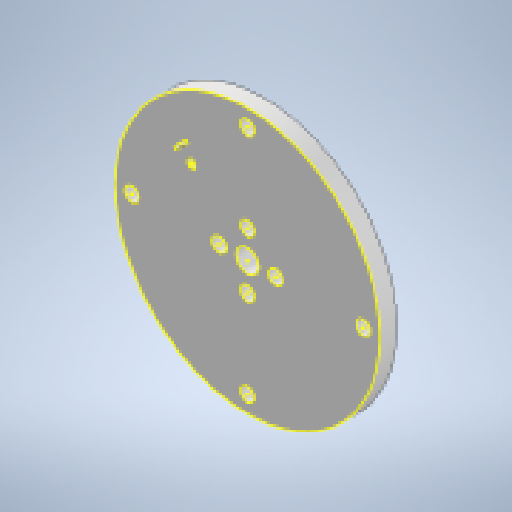
# Autodesk Inventor part: base gear base plate
Saved by Autodesk Inventor 2025 (Build 290162000, 162)
## iProperties
Created: 2025-04-03
Part Number: base gear base plate
Material: 一般
Document SubType Name: Modeling
Designer: gavin
Density: 1 g/cm^3
Appearance: 預設
Author: gavin
Autodesk Inventor part; units mm, degrees
ref_plane "YZ Plane" through (0, 0, 0) normal (1, 0, 0) x (0, 1, 0)
ref_plane "XZ Plane" through (0, 0, 0) normal (0, 1, 0) x (-1, 0, 0)
ref_plane "XY Plane" through (0, 0, 0) normal (0, 0, 1) x (1, 0, 0)
sketch "草圖1" plane through (0, 0, 0) normal (0, 0, 1) x (1, 0, 0)
  circle A0 centre (0, 0) radius 47 projected
  circle A1 centre (40.0673, -8.6957) radius 2.5 construction
  circle A2 centre (-8.6957, -40.0673) radius 2.5 construction
  circle A3 centre (-40.0673, 8.6957) radius 2.5 construction
  circle A4 centre (8.6957, 40.0673) radius 2.5 construction
  circle A5 centre (0, 0) radius 41 construction
  circle A6 centre (41, 0) radius 2.5
  circle A7 centre (0, 41) radius 2.5
  circle A8 centre (-41, 0) radius 2.5
  circle A9 centre (0, -41) radius 2.5
  point P0 (0, 0)
  dimension "d11" = 5
  dimension "d14" = 360
  constraints: 5 centre point, 2 point on circle, 1 coincident, 9 other
  measures "d11" diameter of A6
extrude "擠出1" add sketch "草圖1" along normal blind 6
sketch "草圖3" plane through (0, 0, 6) normal (0, 0, 1) x (1, 0, 0)
  circle A0 centre (0, 0) radius 4
  dimension "d4" = 8
  constraints: 1 centre point, 1 coincident
  measures "d4" diameter of A0
extrude "擠出3" cut sketch "草圖3" against normal through all
sketch "草圖6" plane through (0, 0, 6) normal (0, 0, 1) x (1, 0, 0)
  circle A0 centre (9.4848, 3.1685) radius 2.5 construction
  circle A1 centre (-9.4848, -3.1685) radius 2.5 construction
  circle A2 centre (3.1685, -9.4848) radius 2.5 construction
  circle A3 centre (-3.1685, 9.4848) radius 2.5 construction
  circle A4 centre (0, 0) radius 21 projected
  circle A5 centre (0, 0) radius 4 projected
  circle A6 centre (0, 0) radius 10 construction
  circle A7 centre (10, 0) radius 2.5
  circle A8 centre (0, 10) radius 2.5
  circle A9 centre (-10, 0) radius 2.5
  circle A10 centre (0, -10) radius 2.5
  point P0 (0, 0)
  dimension "d16" = 5
  dimension "d19" = 360
  constraints: 5 centre point, 2 point on circle, 1 coincident, 9 other
  measures "d16" diameter of A7
extrude "擠出5" cut sketch "草圖6" against normal through all contours A7 | A8 | A9 | A10
sketch "草圖10" plane through (0, 0, 6) normal (0, 0, 1) x (1, 0, 0)
  circle A0 centre (-19.8414, 19.8414) radius 1.5
  line L0 (-21.9203, 26.163) -> (-26.163, 21.9203)
  line L1 (-26.163, 21.9203) -> (-25.4983, 21.2556)
  line L2 (-25.4983, 21.2556) -> (-21.2556, 25.4983)
  line L3 (-21.2556, 25.4983) -> (-21.9203, 26.163)
  line L4 (0, 0) -> (-33.234, 33.234) construction
  line L5 (0, 0) -> (18.5986, 0) construction
  circle A1 centre (0, 0) radius 47 projected
  point P0 (-23.377, 23.377)
  dimension "d30" = 3
  dimension "d31" = 0.94
  dimension "d35" = 5
  dimension "d38" = 135
  dimension "d39" = 6
  dimension "d40" = 34
  constraints: 12 end point, 2 parallel, 2 point on line, 1 centre point, 1 horizontal, 1 midpoint, 1 perpendicular, 2 other
  measures "d30" diameter of A0
  measures "d31" distance of L2.end L0.start
  measures "d35" distance from line of L2 A0.centre
  measures "d38" angle of L5 L4
  measures "d39" distance of L0.start L0.end
  measures "d40" distance from line of point (0, 0) L0
extrude "擠出7" cut sketch "草圖10" against normal through all contours A0 | L3 L2 L1 L0
sketch "草圖11" plane through (0, 0, 6) normal (0, 0, 1) x (1, 0, 0)
  circle A0 centre (-19.8414, 19.8414) radius 1.5 projected
  line L0 (-21.2556, 25.4983) -> (-25.4983, 21.2556) projected
  line L1 (-25.4983, 21.2556) -> (-26.163, 21.9203) projected
  line L2 (-26.163, 21.9203) -> (-21.9203, 26.163) projected
  line L3 (-21.9203, 26.163) -> (-21.2556, 25.4983) projected
  circle A1 centre (-10, 0) radius 2.5 projected
  circle A2 centre (0, 10) radius 2.5 projected
  circle A3 centre (0, -10) radius 2.5 projected
  circle A4 centre (10, 0) radius 2.5 projected
  circle A5 centre (0, 0) radius 4 projected
  circle A6 centre (0, 0) radius 47 projected
  circle A7 centre (0, -41) radius 2.5 projected
  circle A8 centre (-41, 0) radius 2.5 projected
  circle A9 centre (0, 41) radius 2.5 projected
  circle A10 centre (41, 0) radius 2.5 projected
